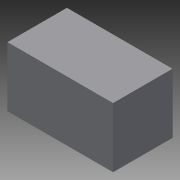
# Autodesk Inventor part: micro
Saved by Autodesk Inventor 2013 (Build 170138000, 138)
## iProperties
Created: 2015-10-02
Part Number: micro
Material: Generic
Document SubType Name: Modeling
Designer: A.Barredo
Density: 1 g/cm^3
Author: A.Barredo
Autodesk Inventor part; units mm, degrees
ref_plane "YZ Plane" through (0, 0, 0) normal (1, 0, 0) x (0, 1, 0)
ref_plane "XZ Plane" through (0, 0, 0) normal (0, 1, 0) x (-1, 0, 0)
ref_plane "XY Plane" through (0, 0, 0) normal (0, 0, 1) x (1, 0, 0)
sketch "Sketch1" plane through (0, 0, 0) normal (0, 1, 0) x (-1, 0, 0)
  line L0 (-4.1439, 2.6989) -> (44.3561, 2.6989)
  line L1 (44.3561, 2.6989) -> (44.3561, -24.8011)
  line L2 (44.3561, -24.8011) -> (-4.1439, -24.8011)
  line L3 (-4.1439, -24.8011) -> (-4.1439, 2.6989)
  point P0 (0, 0)
  dimension "d0" = 48.5
  dimension "d1" = 27.5
  constraints: 8 end point, 2 parallel, 1 horizontal, 1 perpendicular
  measures "d0" distance of L1.end L2.end
  measures "d1" distance of L0.end L1.end
extrude "Extrusion1" add sketch "Sketch1" along normal blind 27.3
body "Solid1"
